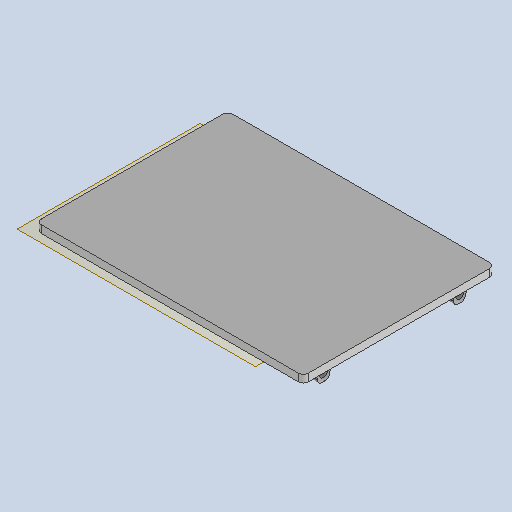
# Autodesk Inventor part: Box_Arduino_Oben_2
Saved by Autodesk Inventor 2024 (Build 280153000, 153)
## iProperties
Created: 2024-02-04
Part Number: Box_Arduino_Oben_2
Material: Generisch
Document SubType Name: Modeling
Designer: Pavel Povolni
Density: 1 g/cm^3
Appearance: Vorgabe
Author: Pavel Povolni
Autodesk Inventor part; units mm, degrees
ref_plane "YZ Plane" through (0, 0, 0) normal (1, 0, 0) x (0, 1, 0)
ref_plane "XZ Plane" through (0, 0, 0) normal (0, 1, 0) x (-1, 0, 0)
ref_plane "XY Plane" through (0, 0, 0) normal (0, 0, 1) x (1, 0, 0)
ref_plane "Arbeitsebene1" through (0, 0, 0) normal (0, 0, 1) x (1, 0, 0)
sketch "Skizze1" plane through (0, 0, 0) normal (0, 0, 1) x (1, 0, 0)
  arc A0 (63, -2) -> (61, 0) centre (61, -2) ccw projected
  line L0 (61, 0) -> (60, 0) projected
  line L1 (60, 0) -> (60, -30) projected
  line L2 (60, -30) -> (-40, -30) projected
  line L3 (-40, -30) -> (-40, 40) projected
  line L4 (-40, 40) -> (60, 40) projected
  line L5 (60, 40) -> (60, 10) projected
  line L6 (60, 10) -> (61, 10) projected
  arc A1 (61, 10) -> (63, 12) centre (61, 12) ccw projected
  line L7 (63, 12) -> (63, 41) projected
  arc A2 (63, 41) -> (61, 43) centre (61, 41) ccw projected
  line L8 (61, 43) -> (-41, 43) projected
  arc A3 (-41, 43) -> (-43, 41) centre (-41, 41) ccw projected
  line L9 (-43, 41) -> (-43, -31) projected
  arc A4 (-43, -31) -> (-41, -33) centre (-41, -31) ccw projected
  line L10 (-41, -33) -> (61, -33) projected
  arc A5 (61, -33) -> (63, -31) centre (61, -31) ccw projected
  line L11 (63, -31) -> (63, -2) projected
  line L12 (63, 12) -> (63, -2)
  point P0 (0, 0)
  constraints: 2 end point, 2 point on circle, 1 vertical
extrude "Extrusion1" add sketch "Skizze1" along normal blind 3
sketch "Skizze2" plane through (0, 0, 0) normal (0, 0, -1) x (-1, 0, 0)
  line L0 (40, -30) -> (-60, -30) construction
  line L1 (-60, -30) -> (-60, 40) construction
  line L2 (-60, 40) -> (40, 40) construction
  line L3 (40, 40) -> (40, -30) construction
  line L4 (40, -24.5) -> (37, -24.5)
  line L5 (37, -24.5) -> (37, -19.5)
  line L6 (37, -19.5) -> (40, -19.5)
  line L7 (40, -19.5) -> (40, -24.5)
  line L8 (40, 29.5) -> (37, 29.5)
  line L9 (37, 29.5) -> (37, 34.5)
  line L10 (37, 34.5) -> (40, 34.5)
  line L11 (40, 34.5) -> (40, 29.5)
  line L12 (-60, -24.5) -> (-57, -24.5)
  line L13 (-57, -24.5) -> (-57, -19.5)
  line L14 (-57, -19.5) -> (-60, -19.5)
  line L15 (-60, -19.5) -> (-60, -24.5)
  line L16 (-60, 29.5) -> (-57, 29.5)
  line L17 (-57, 29.5) -> (-57, 34.5)
  line L18 (-57, 34.5) -> (-60, 34.5)
  line L19 (-60, 34.5) -> (-60, 29.5)
  line L20 (37, -22) -> (40, -22) construction
  line L21 (37, 32) -> (40, 32) construction
  point P0 (38.5, -22)
  dimension "d2" = 3
  dimension "d3" = 5
  dimension "d4" = 8
  dimension "d5" = 8
  constraints: 36 end point, 8 parallel, 6 point on line, 5 midpoint, 4 equal length, 4 horizontal, 4 perpendicular, 2 collinear
  measures "d2" distance of L4.start L4.end
  measures "d3" distance of L4.end L5.end
  measures "d4" distance from line of point (38.5, -22) L0
  measures "d5" distance between parallel lines of L2 L21
extrude "Extrusion2" add sketch "Skizze2" along normal blind 6
sketch "Skizze4" plane through (0, 0, 0) normal (0, 0, -1) x (-1, 0, 0)
  line L0 (-60, 40) -> (40, 40) projected
  line L1 (40, -30) -> (-60, -30) projected
  line L2 (-9.7574, 40) -> (-9.7574, 38)
  line L3 (-9.7574, 38) -> (-29.7574, 38)
  line L4 (-29.7574, 38) -> (-29.7574, 40)
  line L5 (-9.7574, -30) -> (-9.7574, -28)
  line L6 (-9.7574, -28) -> (-29.7574, -28)
  line L7 (-29.7574, -28) -> (-29.7574, -30)
  point P0 (0, 0)
  dimension "d10" = 2
  dimension "d11" = 20
  constraints: 12 end point, 4 perpendicular, 4 point on line, 2 collinear, 1 horizontal, 1 parallel
  measures "d10" distance of L2.start L2.end
  measures "d11" distance of L2.end L3.end
extrude "Extrusion3" add sketch "Skizze4" along normal blind 2
fillet "Rundung1" radius 4 8 edges at (-38.5, 34.5, 0) (-38.5, 29.5, 0) (-38.5, -24.5, 0) (-38.5, -19.5, 0) (58.5, 34.5, 0) (58.5, -19.5, 0) (58.5, 29.5, 0) (58.5, -24.5, 0)
sketch "Skizze5" plane through (60, 29.5, -6) normal (1, 0, 0) x (0, 0, -1)
  circle A0 centre (-3, 2.5) radius 1.55 projected
  circle A1 centre (-3, -51.5) radius 1.55 projected
  point P0 (-6, -29.5)
extrude "Extrusion4" cut sketch "Skizze5" against normal through all
fillet "Rundung2" radius 2 8 edges at (58.5, 29.5, -6) (58.5, 34.5, -6) (58.5, -24.5, -6) (58.5, -19.5, -6) (-38.5, 29.5, -6) (-38.5, 34.5, -6) (-38.5, -24.5, -6) (-38.5, -19.5, -6)
